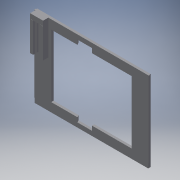
# Autodesk Inventor part: Bovenplaat Frame 2.3
Saved by Autodesk Inventor 2018.3 (Build 223284000, 284)
## iProperties
Created: 2020-12-10
Part Number: Bovenplaat Frame 2.3
Material: Generic
Document SubType Name: Modeling
Designer: daanv
Density: 1 g/cm^3
Appearance: Default
Author: daanv
Autodesk Inventor part; units mm, degrees
ref_plane "YZ Plane" through (0, 0, 0) normal (1, 0, 0) x (0, 1, 0)
ref_plane "XZ Plane" through (0, 0, 0) normal (0, 1, 0) x (-1, 0, 0)
ref_plane "XY Plane" through (0, 0, 0) normal (0, 0, 1) x (1, 0, 0)
sketch "Sketch1" plane through (0, 0, 0) normal (0, 0, 1) x (1, 0, 0)
  line L0 (0, 0) -> (126.5, 0)
  line L1 (126.5, 0) -> (126.5, 2.8)
  line L2 (126.5, 2.8) -> (0, 2.8)
  line L3 (0, 2.8) -> (0, 0)
  dimension "d0" = 126.5
  dimension "d1" = 2.8
  constraints: 8 end point, 2 parallel, 1 horizontal, 1 perpendicular
  measures "d0" distance of L2.end L1.end
  measures "d1" distance of L0.end L1.end
extrude "Extrusion1" add sketch "Sketch1" along normal blind 90
sketch "Sketch2" plane through (0, 0, 90) normal (0, 0, 1) x (1, 0, 0)
  line L0 (126.5, 0) -> (126.5, 2.8) projected
  line L1 (0, 2.8) -> (0, 0) projected
  line L2 (126.5, 0.15) -> (127.2, 0.15)
  line L3 (127.2, 0.15) -> (127.2, 1.55)
  line L4 (127.2, 1.55) -> (126.5, 1.55)
  line L5 (126.5, 1.55) -> (126.5, 0.15)
  line L6 (0, 0.15) -> (-0.7, 0.15)
  line L7 (-0.7, 0.15) -> (-0.7, 1.55)
  line L8 (-0.7, 1.55) -> (0, 1.55)
  line L9 (0, 1.55) -> (0, 0.15)
  line L10 (126.5, 2.8) -> (0, 2.8) projected
  dimension "d4" = 0.7
  dimension "d5" = 1.4
  dimension "d6" = 0.7
  dimension "d7" = 1.4
  dimension "d17" = 1.25
  dimension "d18" = 1.25
  constraints: 16 end point, 4 parallel, 2 horizontal, 2 perpendicular, 2 point on line
  measures "d4" distance of L4.end L3.end
  measures "d5" distance of L3.end L2.end
  measures "d6" distance of L7.end L8.end
  measures "d7" distance of L6.end L7.end
  measures "d17" distance between parallel lines of L10 L8
  measures "d18" distance between parallel lines of L10 L4
extrude "Extrusion2" add sketch "Sketch2" against normal blind 85
sketch "Sketch3" plane through (0, 0, 0) normal (0, -1, 0) x (1, 0, 0)
  line L0 (0, 90) -> (126.5, 90) projected
  line L1 (0, 0) -> (0, 90) projected
  line L2 (0.6, 90) -> (15.1, 90)
  line L3 (15.1, 90) -> (15.1, 84.58)
  line L4 (15.1, 84.58) -> (0.6, 84.58)
  line L5 (0.6, 84.58) -> (0.6, 90)
  dimension "d12" = 14.5
  dimension "d13" = 5.42
  dimension "d14" = 0.6
  constraints: 8 end point, 2 parallel, 1 horizontal, 1 perpendicular, 1 point on line
  measures "d12" distance of L3.end L4.end
  measures "d13" distance of L2.end L3.end
  measures "d14" distance between parallel lines of L1 L5
extrude "Extrusion3" add sketch "Sketch3" along normal blind 5.72
sketch "Sketch4" plane through (0, 0, 0) normal (0, -1, 0) x (1, 0, 0)
  line L0 (15.1, 90) -> (15.1, 84.58) projected
  line L1 (15.1, 84.58) -> (0.6, 84.58) projected
  line L2 (0.6, 84.58) -> (0.6, 90) projected
  line L3 (0, 90) -> (0.6, 90) projected
  line L4 (0, 0) -> (0, 90) projected
  line L5 (0, 0) -> (126.5, 0) projected
  line L6 (126.5, 0) -> (126.5, 90) projected
  line L7 (15.1, 90) -> (126.5, 90) projected
extrude "Extrusion4" cut sketch "Sketch4" against normal blind 0.15
sketch "Sketch5" plane through (0, 0.15, 0) normal (0, -1, 0) x (1, 0, 0)
  line L0 (0.6, 84.58) -> (15.1, 84.58) projected
  line L1 (0.6, 84.58) -> (2.6, 84.58)
  line L2 (2.6, 84.58) -> (2.6, 51.58)
  line L3 (2.6, 51.58) -> (0.6, 51.58)
  line L4 (0.6, 51.58) -> (0.6, 84.58)
  line L5 (15.1, 84.58) -> (13.1, 84.58)
  line L6 (13.1, 84.58) -> (13.1, 51.58)
  line L7 (13.1, 51.58) -> (15.1, 51.58)
  line L8 (15.1, 51.58) -> (15.1, 84.58)
  dimension "d21" = 33
  dimension "d22" = 2
  dimension "d23" = 2
  dimension "d24" = 10.5
  constraints: 16 end point, 4 parallel, 2 horizontal, 2 perpendicular, 1 point on line
  measures "d21" distance of L1.end L2.end
  measures "d22" distance of L6.end L7.end
  measures "d23" distance of L2.end L3.end
  measures "d24" distance between parallel lines of L6 L2
extrude "Extrusion5" add sketch "Sketch5" along normal blind 6
sketch "Sketch6" plane through (2.6, 0.15, 51.58) normal (0, 0, -1) x (-1, 0, 0)
  line L0 (0, 0) -> (0, -6) projected
  line L1 (2, -6) -> (0, -6) projected
  line L2 (0, -2) -> (-1.5, -2)
  line L3 (-1.5, -2) -> (-1.5, 0)
  line L4 (-1.5, 0) -> (0, 0)
  line L5 (0, 0) -> (0, -2)
  point P0 (2.6, -0.15)
  dimension "d27" = 4
  dimension "d28" = 2
  dimension "d29" = 1.5
  constraints: 8 end point, 2 parallel, 1 horizontal, 1 perpendicular, 1 point on line
  measures "d27" distance between parallel lines of L1 L2
  measures "d28" distance of L2.end L3.end
  measures "d29" distance between parallel lines of L5 L3
extrude "Extrusion6" add sketch "Sketch6" against normal blind 33
sketch "Sketch7" plane through (2.6, -5.85, 51.58) normal (0, 0, -1) x (-1, 0, 0)
  line L0 (0, 4) -> (1.65, 4)
  line L1 (1.65, 4) -> (1.65, 2.4)
  line L2 (1.65, 2.4) -> (0, 2.4)
  line L3 (0, 2.4) -> (0, 4)
  point P0 (2.6, 5.85)
  dimension "d32" = 1.65
  dimension "d33" = 1.6
  constraints: 8 end point, 2 parallel, 1 horizontal, 1 perpendicular
  measures "d32" distance of L1.end L2.end
  measures "d33" distance of L0.end L1.end
extrude "Extrusion7" cut sketch "Sketch7" against normal blind 33
sketch "Sketch8" plane through (15.1, 0.15, 51.58) normal (0, 0, -1) x (-1, 0, 0)
  line L0 (2, 0) -> (3.5, 0)
  line L1 (3.5, 0) -> (3.5, -2)
  line L2 (3.5, -2) -> (2, -2)
  line L3 (2, -2) -> (2, 0)
  point P0 (15.1, -0.15)
  dimension "d36" = 1.5
  dimension "d37" = 2
  constraints: 8 end point, 2 parallel, 1 horizontal, 1 perpendicular
  measures "d36" distance of L1.end L2.end
  measures "d37" distance between parallel lines of L0 L2
extrude "Extrusion8" add sketch "Sketch8" against normal blind 33
sketch "Sketch9" plane through (15.1, -5.85, 51.58) normal (0, 0, -1) x (-1, 0, 0)
  line L0 (2, 4) -> (0.35, 4)
  line L1 (0.35, 4) -> (0.35, 2.4)
  line L2 (0.35, 2.4) -> (2, 2.4)
  line L3 (2, 2.4) -> (2, 4)
  point P0 (15.1, 5.85)
  dimension "d40" = 1.65
  dimension "d41" = 1.6
  constraints: 8 end point, 2 parallel, 1 horizontal, 1 perpendicular
  measures "d40" distance of L2.end L1.end
  measures "d41" distance of L1.end L0.end
extrude "Extrusion9" cut sketch "Sketch9" against normal blind 33
sketch "Sketch10" plane through (13.1, -5.85, 51.58) normal (-1, 0, 0) x (0, 0, 1)
  line L0 (33, 2.4) -> (0, 2.4) projected
  line L1 (0, 2.4) -> (0, 0) projected
  line L2 (33, 0) -> (0, 0) projected
  line L3 (33, 0.13) -> (33, 0) projected
  line L4 (33, 2.4) -> (33, 0.13) projected
  point P0 (-51.58, 5.85)
extrude "Extrusion10" add sketch "Sketch10" along normal blind 1.5
sketch "Sketch11" plane through (2.6, -5.85, 84.58) normal (1, 0, 0) x (0, 0, -1)
  line L0 (33, 2.4) -> (0, 2.4) projected
  line L1 (0, 0.13) -> (0, 2.4) projected
  line L2 (0, 0.13) -> (0, 0) projected
  line L3 (33, 0) -> (0, 0) projected
  line L4 (33, 2.4) -> (33, 0) projected
  point P0 (84.58, 5.85)
extrude "Extrusion11" add sketch "Sketch11" along normal blind 1.5
sketch "Sketch12" plane through (0, 2.8, 0) normal (0, 1, 0) x (1, 0, 0)
  line L0 (18.25, -10) -> (108.25, -10)
  line L1 (108.25, -10) -> (108.25, -80)
  line L2 (108.25, -80) -> (18.25, -80)
  line L3 (18.25, -80) -> (18.25, -10)
  line L4 (126.5, 0) -> (0, 0) projected
  line L5 (0, 0) -> (0, -90) projected
  line L6 (126.5, -90) -> (0, -90) projected
  line L7 (126.5, 0) -> (126.5, -90) projected
  line L8 (47.32, -80) -> (63.75, -80)
  line L9 (63.75, -80) -> (63.75, -85)
  line L10 (63.75, -85) -> (47.32, -85)
  line L11 (47.32, -85) -> (47.32, -80)
  line L12 (47.32, -10) -> (63.75, -10)
  line L13 (63.75, -10) -> (63.75, -5)
  line L14 (63.75, -5) -> (47.32, -5)
  line L15 (47.32, -5) -> (47.32, -10)
  dimension "d51" = 90
  dimension "d52" = 70
  dimension "d55" = 18.25
  dimension "d56" = 18.25
  dimension "d57" = 10
  dimension "d58" = 10
  dimension "d59" = 16.43
  dimension "d60" = 5
  dimension "d61" = 29.07
  dimension "d67" = 5
  dimension "d68" = 29.07
  constraints: 24 end point, 6 parallel, 3 horizontal, 3 perpendicular, 2 point on line
  measures "d51" distance of L1.end L2.end
  measures "d52" distance of L0.end L1.end
  measures "d55" distance between parallel lines of L5 L3
  measures "d56" distance between parallel lines of L7 L1
  measures "d57" distance between parallel lines of L4 L0
  measures "d58" distance between parallel lines of L6 L2
  measures "d59" distance of L9.end L10.end
  measures "d60" distance of L8.end L9.end
  measures "d61" distance between parallel lines of L3 L11
  measures "d67" distance of L13.end L12.end
  measures "d68" distance between parallel lines of L3 L15
extrude "Extrusion13" cut sketch "Sketch12" against normal up to next contours L0 L1 L2 L3 | L15 L14 L13 L0 | L2 L9 L10 L11
chamfer "Chamfer1" distance 1.2 angle 60 1 edges at (47.32, 2.8, 82.5) measured on face at (6.0833, 2.8, 56.6667)
chamfer "Chamfer2" distance 1.2 angle 60 1 edges at (47.32, 2.8, 7.5) measured on face at (6.0833, 2.8, 56.6667)
body "Solid1"
